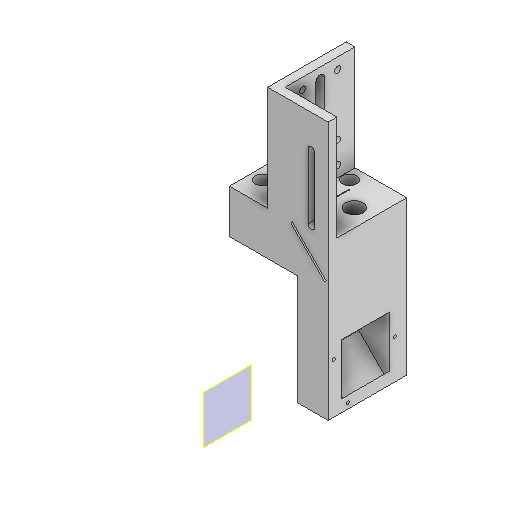
# Autodesk Inventor part: TIRFImager_Laserbase_v1
Saved by Autodesk Inventor 2024.1 (Build 281209000, 209)
## iProperties
Created: 2022-05-21
Part Number: TIRFImager_Laserbase_v1
Material: Generisch
Document SubType Name: Modeling
Designer: diederichbenedict
Density: 1 g/cm^3
Appearance: Vorgabe
Author: diederichbenedict
Autodesk Inventor part; units mm, degrees
ref_plane "YZ Plane" through (0, 0, 0) normal (1, 0, 0) x (0, 1, 0)
ref_plane "Arbeitsebene1" through (49.1253, 12.3022, -77.9087) normal (-1, 0, 0) x (0, -1, 0)
sketch "Skizze1" plane through (49.1253, 9.0962, -77.9087) normal (1, 0, 0) x (0, 1, 0)
  line L0 (2.603, 4) -> (2.603, 19.5) construction
  line L1 (2.603, 19.5) -> (-10.897, 19.5) construction
  line L2 (-10.897, 19.5) -> (-10.897, 4) construction
  line L3 (-10.897, 4) -> (2.603, 4) construction
  circle A0 centre (6.603, 29.5) radius 1 construction
  circle A1 centre (-13.897, 23) radius 1 construction
  circle A2 centre (1.603, 1.5) radius 1 construction
  arc A3 (8.303, 27.8555) -> (9.303, 28.8555) centre (8.303, 28.8555) ccw construction
  line L4 (8.303, 27.8555) -> (5.5653, 27.8555) construction
  arc A4 (5.5653, 27.8555) -> (4.5653, 26.8555) centre (5.5653, 26.8555) ccw construction
  line L5 (4.5653, 26.8555) -> (4.5653, 0) construction
  arc A5 (3.5653, -1) -> (4.5653, 0) centre (3.5653, 0) ccw construction
  line L6 (3.5653, -1) -> (1, -1) construction
  arc A6 (0, 0) -> (1, -1) centre (1, 0) ccw construction
  line L7 (0, 0) -> (0, 1) construction
  arc A7 (0, 1) -> (-1, 2) centre (-1, 1) ccw construction
  line L8 (-1, 2) -> (-12.5347, 2) construction
  line L9 (-12.5347, 2) -> (-12.5347, 20.4723) construction
  arc A8 (-12.5347, 20.4723) -> (-13.5347, 21.4723) centre (-13.5347, 20.4723) ccw construction
  line L10 (-13.5347, 21.4723) -> (-15.397, 21.4723) construction
  arc A9 (-16.397, 22.4723) -> (-15.397, 21.4723) centre (-15.397, 22.4723) ccw construction
  line L11 (-16.397, 22.4723) -> (-16.397, 32) construction
  line L12 (-16.397, 32) -> (9.303, 32) construction
  line L13 (9.303, 32) -> (9.303, 28.8555) construction
  line L14 (-10.897, 4) -> (10.603, 4)
  line L15 (10.603, 4) -> (10.603, 26)
  line L16 (10.603, 26) -> (-10.897, 26)
  line L17 (-10.897, 26) -> (-10.897, 4)
  circle A10 centre (1.603, 1.5) radius 0.75
  circle A11 centre (6.603, 29.5) radius 0.75
  circle A12 centre (-13.897, 23) radius 0.75
  line L18 (71.478, -4) -> (23.478, -4) projected
  line L19 (71.478, 28) -> (23.478, 28) projected
  line L20 (-16.397, -4) -> (13.603, -4)
  line L21 (13.603, -4) -> (13.603, 32)
  line L22 (13.603, 32) -> (-16.397, 32)
  line L23 (-16.397, 32) -> (-16.397, -4)
  point P0 (-9.0962, 77.9087)
  dimension "d0" = 22
  dimension "d1" = 1.5
  dimension "d2" = 1.5
  dimension "d3" = 1.5
  dimension "d4" = 30
  constraints: 16 end point, 4 parallel, 3 centre point, 3 coincident, 2 horizontal, 2 perpendicular
  measures "d0" distance of L15.end L14.end
  measures "d1" diameter of A10
  measures "d2" diameter of A11
  measures "d3" diameter of A12
  measures "d4" distance of L22.end L21.end
extrude "Extrusion1" add sketch "Skizze1" against normal blind 14
sketch "Skizze2" plane through (49.1253, 22.6992, -81.9087) normal (0, 0, -1) x (1, 0, 0)
  line L0 (-14, 30) -> (-14, 0) projected
  line L1 (-45.2, -6.375) -> (-15.2, -6.375) projected
  line L2 (-15.2, -20.375) -> (-15.2, -6.375) projected
  line L3 (-45.2, -20.375) -> (-15.2, -20.375) projected
  line L4 (-45.2, -20.375) -> (-45.2, -6.375) projected
  circle A0 centre (-30.2, -12.225) radius 2.75 projected
  line L5 (0, 0) -> (-14, 0)
  line L6 (-14, 0) -> (-14, -40.375)
  line L7 (-14, -40.375) -> (0, -40.375)
  line L8 (0, -40.375) -> (0, 0)
  line L9 (-14, -40.375) -> (-45.2, -40.375)
  line L10 (-45.2, -40.375) -> (-45.2, -20.375)
  line L11 (-45.2, -20.375) -> (-14, -20.375)
  line L12 (-14, -20.375) -> (-14, -40.375)
  point P0 (-49.1253, 22.6992)
  dimension "d39" = 20
  constraints: 16 end point, 4 parallel, 2 horizontal, 2 perpendicular
  measures "d39" distance between parallel lines of L9 L3
extrude "Extrusion2" add sketch "Skizze2" against normal up to surface (36 mm away) contours L3 L11 L6 L9 L10 | L6 L5 L8 L7
sketch "Skizze4" plane through (49.1253, -7.3008, -45.9087) normal (0, 0, 1) x (-1, 0, 0)
  line L0 (0, -70.375) -> (23.7, -70.375)
  line L1 (7.7, -103.375) -> (7.7, -65.3352) construction
  line L2 (9.2, -103.375) -> (9.2, -73.375)
  line L3 (6.2, -73.375) -> (6.2, -103.375)
  arc A0 (6.2, -103.375) -> (9.2, -103.375) centre (7.7, -103.375) ccw
  arc A1 (9.2, -73.375) -> (6.2, -73.375) centre (7.7, -73.375) ccw
  circle A2 centre (7.7, -75.375) radius 1.4
  line L4 (23.7, -118.375) -> (-8.3, -118.375)
  line L5 (23.7, -70.375) -> (0, -70.375)
  line L6 (0, -70.375) -> (0, -118.375)
  line L7 (0, -118.375) -> (23.7, -118.375)
  line L8 (23.7, -118.375) -> (23.7, -70.375)
  point P0 (49.1253, -7.3008)
  point P1 (7.7, -84.3551)
  point P2 (6.2, -70.375)
  point P3 (9.2, -70.375)
  dimension "d13" = 3
  dimension "d40" = 0
  dimension "d62" = 15
  dimension "d63" = 30
  constraints: 19 end point, 4 point on circle, 4 tangent, 3 centre point, 3 horizontal, 3 parallel, 1 coincident, 1 midpoint, 1 perpendicular, 1 point on line, 1 vertical, 4 other
  measures "d13" diameter of A1
  measures "d40" horizontal distance of L1.start A2.centre
  measures "d62" distance from line of L1.start L4
  measures "d63" distance of A1.centre L1.start
ref_plane "Arbeitsebene2" through (41.1253, -49.1758, -49.9087) normal (0, 0, 1) x (1, 0, 0)
ref_plane "Arbeitsebene3" through (40.8253, -69.6758, -49.9087) normal (0, 0, 1) x (1, 0, 0)
extrude "Extrusion4" add sketch "Skizze4" against normal up to surface (4 mm away) contours L0 L8 L4 L6
sketch "Skizze6" plane through (49.1253, 63.0742, -81.9087) normal (0, 1, 0) x (-1, 0, 0)
  circle A0 centre (8, 16) radius 2.5 projected
  circle A1 centre (8, 16) radius 4
  point P0 (49.1253, 81.9087)
  dimension "d19" = 8
  constraints: 1 centre point, 1 coincident
  measures "d19" diameter of A1
extrude "Extrusion6" cut sketch "Skizze6" against normal blind 42 contours A0 | A1
sketch "Skizze7" plane through (49.1253, -7.3008, -45.9087) normal (0, 0, 1) x (-1, 0, 0)
  line L0 (4, -19) -> (12, -19) projected
  line L1 (0.1, -13) -> (-7.6, -13)
  line L2 (-7.6, -13) -> (8, -13)
  line L3 (8, -13) -> (8, -19)
  line L4 (0, -5) -> (14, -19)
  line L5 (0, -5) -> (19.799, -5) construction
  line L6 (14, 0) -> (14, -50.375) projected
  line L7 (0, 0) -> (0, -25.7) projected
  line L8 (0, -5.5) -> (14, -5.5) projected
  line L9 (14, -5.5) -> (14, -27) projected
  line L10 (0.5, -5.5) -> (14, -5.5)
  line L11 (14, -19) -> (14, -5.5)
  line L12 (4.7426, -5.5) -> (14, -14.7574)
  point P0 (49.1253, -7.3008)
  point P1 (15, -28)
  point P2 (14, -25)
  point P3 (4.7426, -5.5)
  point P4 (14, -30)
  point P5 (14, -39.875)
  dimension "d22" = 45
  dimension "d23" = 3
  constraints: 16 end point, 6 point on line, 4 horizontal, 1 equal length, 1 midpoint, 1 perpendicular, 1 vertical, 4 other
  measures "d22" angle of L4 L5
  measures "d23" distance between parallel lines of L12 L4
extrude "Extrusion7" add sketch "Skizze7" against normal up to surface (28 mm away) contours L8 L6 L12
sketch "Skizze9" plane through (49.1253, 19.6992, -51.9087) normal (0, -1, 0) x (-1, 0, 0)
  line L0 (0, 22) -> (14, 22) projected
  line L1 (0, 0) -> (0, 22) projected
  line L2 (0, 0) -> (14, 0) projected
  line L3 (15, -6) -> (15, 30) projected
  line L4 (14, 0) -> (15, 0)
  line L5 (15, 0) -> (15, 22)
  line L6 (15, 22) -> (14, 22)
  line L7 (14, 22) -> (14, 0)
  line L8 (14, 22) -> (14, 0) projected
  point P0 (49.1253, -51.9087)
  constraints: 8 end point, 2 parallel, 1 horizontal, 1 perpendicular, 1 point on line
extrude "Extrusion9" cut sketch "Skizze9" against normal blind 2
sketch "Skizze10" plane through (44.3827, -1.8008, -51.9087) normal (0.7071, 0.7071, 0) x (0.7071, -0.7071, 0)
  line L0 (0, 0) -> (-13.0919, 0) projected
  line L1 (0, 22) -> (0, 0) projected
  line L2 (-13.0919, 22) -> (0, 22) projected
  line L3 (-13.0919, 0) -> (-13.0919, 22) projected
  line L4 (3.3536, 22) -> (3.3536, 0) projected
  line L5 (0, 0) -> (3.3536, 0)
  line L6 (3.3536, 0) -> (3.3536, 22)
  line L7 (3.3536, 22) -> (0, 22)
  line L8 (0, 22) -> (0, 0)
  point P0 (-32.6566, -51.9087)
  point P1 (3.3536, 0)
  constraints: 8 end point, 2 parallel, 1 horizontal, 1 perpendicular
extrude "Extrusion10" cut sketch "Skizze10" along normal blind 4
sketch "Skizze11" plane through (49.1253, 63.0742, -81.9087) normal (0, 1, 0) x (-1, 0, 0)
  circle A0 centre (40.2, 26) radius 1.25 projected
  circle A1 centre (40.2, 6) radius 1.25 projected
  circle A2 centre (40.2, 26) radius 1.25 projected
  circle A3 centre (40.2, 6) radius 1.25 projected
  circle A4 centre (20.2, 6) radius 1.25 projected
  circle A5 centre (20.2, 26) radius 1.25 projected
  point P0 (49.1253, 81.9087)
hole "Bohrung1" at (8.9253, 63.0742, -55.9087) at (8.9253, 63.0742, -75.9087) at (28.9253, 63.0742, -55.9087) at (28.9253, 63.0742, -75.9087) direction (0, -1, 0) diameter 3 end through all counterbore diameter 6.5 counterbore depth 14
sketch "Skizze12" plane through (25.4253, 101.0742, -45.9087) normal (-1, 0, 0) x (0, 0, -1)
  circle A0 centre (12, 23) radius 1.4 projected
  circle A1 centre (20, 23) radius 1.4 projected
  circle A2 centre (28, 33) radius 1.4 projected
  circle A3 centre (20, 33) radius 1.4 projected
  circle A4 centre (20, -5) radius 1.4 projected
  circle A5 centre (28, -5) radius 1.4 projected
  circle A6 centre (12, 33) radius 1.4 projected
  circle A7 centre (28, 23) radius 1.4 projected
  circle A8 centre (12, -5) radius 1.4 projected
  line L0 (36, -10) -> (4, -10) projected
  line L1 (36, -10) -> (36, 38) projected
  line L2 (4, 38) -> (36, 38) projected
  line L3 (4, -10) -> (4, 38) projected
  line L4 (20, 33) -> (20, -5) construction
  line L5 (18, 33) -> (18, -5)
  line L6 (22, -5) -> (22, 33)
  arc A9 (22, 33) -> (18, 33) centre (20, 33) ccw
  arc A10 (18, -5) -> (22, -5) centre (20, -5) ccw
  line L7 (0, -10) -> (4, -10) projected
  line L8 (0, 38) -> (4, 38) projected
  line L9 (0, -10) -> (4, -10)
  line L10 (4, -10) -> (4, 38)
  line L11 (4, 38) -> (0, 38)
  line L12 (0, 38) -> (0, -10)
  point P0 (-45.9087, 101.0742)
  point P1 (20, 14)
  dimension "d50" = 4
  constraints: 16 end point, 4 point on circle, 4 tangent, 3 parallel, 2 centre point, 1 horizontal, 1 midpoint, 1 perpendicular, 1 vertical
  measures "d50" diameter of A10
extrude "Extrusion11" add sketch "Skizze12" along normal blind 4 contours L0 L3 L2 L1 | L7 L12 L8 L3
sketch "Skizze13" plane through (35.1253, -7.3008, -45.9087) normal (0, 0, 1) x (1, 0, 0)
  line L0 (13.1087, 54.9805) -> (-2.4476, 70.5368)
  line L1 (-2.4476, 70.5368) -> (-3.1547, 69.8297)
  line L2 (-3.1547, 69.8297) -> (12.4016, 54.2734)
  line L3 (12.4016, 54.2734) -> (13.1087, 54.9805)
  line L4 (13.1087, 54.9805) -> (-3.1547, 69.8297) construction
  line L5 (-2.4476, 70.5368) -> (12.4016, 54.2734) construction
  line L6 (13.1087, 54.9805) -> (35.1087, 54.9805) construction
  line L7 (6.3, 60.775) -> (6.3, 127.975)
  line L8 (6.3, 60.775) -> (6.3, 49.3956)
  line L9 (6.3, 60.375) -> (-16.5354, 60.375)
  line L10 (0, 0) -> (0, 50.375) projected
  line L11 (14, 0) -> (0, 0) projected
  line L12 (14, 0) -> (14, 118.375) projected
  line L13 (14, 118.375) -> (-13.7, 118.375) projected
  line L14 (-13.7, 70.375) -> (-13.7, 118.375) projected
  line L15 (-31.2, 70.375) -> (-13.7, 70.375) projected
  line L16 (-31.2, 50.375) -> (-31.2, 70.375) projected
  line L17 (0, 50.375) -> (-31.2, 50.375) projected
  line L18 (4.8, 73.375) -> (4.8, 103.375) projected
  arc A0 (7.8, 103.375) -> (4.8, 103.375) centre (6.3, 103.375) ccw projected
  line L19 (7.8, 103.375) -> (7.8, 73.375) projected
  arc A1 (4.8, 73.375) -> (7.8, 73.375) centre (6.3, 73.375) ccw projected
  point P0 (-35.1253, 7.3008)
  dimension "d53" = 22
  dimension "d54" = 135
  dimension "d55" = 1
  dimension "d56" = 20
  dimension "d57" = 10
  constraints: 20 end point, 2 parallel, 2 perpendicular, 2 point on line, 2 vertical, 1 equal length, 1 horizontal, 2 other
  measures "d53" distance of L0.start L0.end
  measures "d54" angle of L6 L0
  measures "d55" distance of L1.end L0.end
  measures "d56" distance between parallel lines of L17 L15
  measures "d57" distance between parallel lines of L9 L15
extrude "Extrusion12" cut sketch "Skizze13" against normal blind 26 contours L3 L2 L8 L7 L0 | L7 L8 L2 L1 L0
sketch "Skizze14" plane through (3.9253, 43.0742, -81.9087) normal (-1, 0, 0) x (0, 0, 1)
  circle A0 centre (16, 11.7142) radius 4 projected
  circle A1 centre (16, 11.7142) radius 7.25
  point P0 (81.9087, -43.0742)
  dimension "d69" = 14.5
  constraints: 1 centre point, 1 coincident
  measures "d69" diameter of A1
extrude "Extrusion13" cut sketch "Skizze14" against normal up to surface contours A0 | A1 surface through (32.6777, 63.236, -45.9087) normal (0.7071, 0.7071, 0)
sketch "Skizze15" plane through (3.9253, 43.0742, -81.9087) normal (-1, 0, 0) x (0, 0, 1)
  line L0 (36, 0) -> (36, 20) projected
  line L1 (0, 20) -> (36, 20) projected
  line L2 (0, 0) -> (0, 20) projected
  line L3 (0, 0) -> (36, 0) projected
  line L4 (36, 3.8984) -> (10, 3.8984) projected
  circle A0 centre (16, 3.8984) radius 1.4
  circle A1 centre (30.7551, 3.8984) radius 1.4
  circle A2 centre (30.7551, 11.7142) radius 1.4
  point P0 (81.9087, -43.0742)
  dimension "d64" = 2.8
  dimension "d65" = 2.8
  dimension "d66" = 2.8
  constraints: 3 centre point, 2 point on line
  measures "d64" diameter of A0
  measures "d65" diameter of A1
  measures "d66" diameter of A2
extrude "Extrusion14" cut sketch "Skizze15" against normal blind 10 contours A0 L4 | L4 A0 | A1 L4 | L4 A1 | A2
